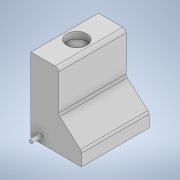
# Autodesk Inventor part: leg
Saved by Autodesk Inventor 2021 (Build 250183000, 183)
## iProperties
Created: 2021-07-04
Part Number: leg
Material: Generic
Document SubType Name: Modeling
Designer: Admin
Density: 1 g/cm^3
Appearance: Default
Author: Admin
Autodesk Inventor part; units mm, degrees
ref_plane "YZ Plane" through (0, 0, 0) normal (1, 0, 0) x (0, 1, 0)
ref_plane "XZ Plane" through (0, 0, 0) normal (0, 1, 0) x (-1, 0, 0)
ref_plane "XY Plane" through (0, 0, 0) normal (0, 0, 1) x (1, 0, 0)
sketch "Sketch18" plane through (0, 0, 0) normal (0, 0, 1) x (1, 0, 0)
  line L0 (0, 0) -> (0, 220)
  line L1 (0, 0) -> (150, 0)
  line L2 (0, 220) -> (82.0223, 220)
  line L3 (82.0223, 220) -> (82.0223, 100)
  line L4 (150, 0) -> (150, 40)
  line L5 (150, 40) -> (82.0223, 100)
  dimension "d72" = 220
  dimension "d73" = 150
  dimension "d74" = 120
  dimension "d75" = 40
  constraints: 12 end point, 2 horizontal, 2 vertical, 1 perpendicular
  measures "d72" distance of L0.start L0.end
  measures "d73" distance of L0.start L1.end
  measures "d74" distance of L2.end L3.end
  measures "d75" distance of L1.end L4.end
extrude "Extrusion9" add sketch "Sketch18" along normal blind 200
sketch "Sketch20" plane through (0, 0, 200) normal (0, 0, 1) x (1, 0, 0)
  circle A0 centre (30, 20) radius 5
  point P0 (0, 0)
  dimension "d81" = 10
  constraints: 1 centre point
  measures "d81" diameter of A0
extrude "Extrusion11" cut sketch "Sketch20" against normal blind 200
fillet "Fillet3" radius 10 3 edges at (82.0223, 220, 100) (82.0223, 100, 100) (150, 40, 100)
sketch "Sketch21" plane through (0, 220, 200) normal (0, 1, 0) x (1, 0, 0)
  circle A0 centre (36, 100) radius 30
  point P0 (0, 200)
  dimension "d85" = 60
  constraints: 1 centre point
  measures "d85" diameter of A0
extrude "Extrusion12" cut sketch "Sketch21" against normal blind 20
sketch "Sketch22" plane through (0, 0, 0) normal (-1, 0, 0) x (0, 0, 1)
  point P0 (0, 0)
sketch "Sketch23" plane through (0, 0, 0) normal (0, 0, -1) x (-1, 0, 0)
  point P0 (0, 0)
sketch "Sketch24" plane through (0, 0, 0) normal (0, 0, -1) x (-1, 0, 0)
  circle A0 centre (-30, 20) radius 5 projected
  circle A1 centre (-30, 20) radius 5
  point P0 (0, 0)
  constraints: 1 centre point, 1 coincident
extrude "Extrusion13" add sketch "Sketch24" along normal blind 30
sketch "Sketch25" plane through (0, 0, 200) normal (0, 0, 1) x (1, 0, 0)
  circle A0 centre (30, 20) radius 5 projected
  circle A1 centre (30, 20) radius 5
  point P0 (0, 0)
  constraints: 1 centre point, 1 coincident
extrude "Extrusion14" add sketch "Sketch25" along normal blind 30
body "Solid5"
